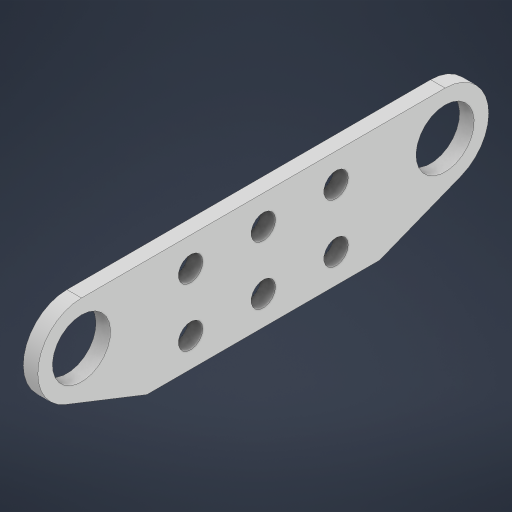
# Autodesk Inventor part: ElevatorCarriageBearingGusset
Saved by Autodesk Inventor 2023 (Build 270158000, 158)
## iProperties
Created: 2023-01-08
Part Number: ElevatorCarriageBearingGusset
Material: Generic
Document SubType Name: Modeling
Designer: Terrence
Density: 1 g/cm^3
Appearance: Default
Author: Terrence
Autodesk Inventor part; units mm, degrees
ref_plane "YZ Plane" through (0, 0, 0) normal (1, 0, 0) x (0, 1, 0)
ref_plane "XZ Plane" through (0, 0, 0) normal (0, 1, 0) x (-1, 0, 0)
ref_plane "XY Plane" through (0, 0, 0) normal (0, 0, 1) x (1, 0, 0)
sketch "Sketch1" plane through (0, 0, 0) normal (1, 0, 0) x (0, 1, 0)
  line L0 (0, 0) -> (25.4, 0)
  line L1 (25.4, 0) -> (25.4, -50.8)
  line L2 (25.4, -50.8) -> (0, -50.8)
  line L3 (0, -50.8) -> (0, 0)
  arc A0 (25.4, 14.2875) -> (7.0144, 17.7826) centre (15.875, 14.2875) ccw
  line L4 (25.4, 0) -> (25.4, 14.2875)
  line L5 (7.0144, 17.7826) -> (0, 0)
  line L6 (15.875, 14.2875) -> (15.875, 0) construction
  circle A1 centre (15.875, 14.2875) radius 14.2875 construction
  line L7 (25.4, -25.4) -> (0, -25.4) construction
  arc A2 (7.0144, -68.5826) -> (25.4, -65.0875) centre (15.875, -65.0875) ccw
  line L8 (25.4, -50.8) -> (25.4, -65.0875)
  line L9 (7.0144, -68.5826) -> (0, -50.8)
  circle A3 centre (15.875, 14.2875) radius 6.35
  circle A4 centre (15.875, -65.0875) radius 6.35
  dimension "d0" = 25.4
  dimension "d1" = 50.8
  dimension "d3" = 19.05
  dimension "d7" = 28.575
  dimension "d8" = 14.2875
  dimension "d11" = 12.7
  constraints: 20 end point, 5 centre point, 4 point on circle, 4 symmetric about line, 2 coincident, 2 midpoint, 2 parallel, 2 perpendicular, 2 tangent, 1 horizontal, 1 point on line, 1 vertical, 2 other
  measures "d0" distance of L1.end L2.end
  measures "d1" distance of L0.end L1.end
  measures "d3" diameter of A0
  measures "d7" diameter of A1
  measures "d8" distance of L6.start L6.end
  measures "d11" diameter of A3
extrude "Extrusion1" add sketch "Sketch1" along normal blind 3.175
sketch "Sketch2" plane through (3.175, 0, 0) normal (1, 0, 0) x (0, 0, -1)
  line L0 (65.0875, 25.4) -> (-14.2875, 25.4) projected
  line L1 (25.4, 25.4) -> (25.4, 0) construction
  line L2 (0, 0) -> (50.8, 0) projected
  line L3 (0, 25.4) -> (50.8, 25.4) construction
  line L4 (50.8, 25.4) -> (50.8, 50.8) construction
  line L5 (50.8, 50.8) -> (0, 50.8) construction
  line L6 (0, 50.8) -> (0, 25.4) construction
  line L7 (3.175, 47.625) -> (47.625, 47.625) construction
  line L8 (47.625, 47.625) -> (47.625, 28.575) construction
  line L9 (47.625, 28.575) -> (3.175, 28.575) construction
  line L10 (3.175, 28.575) -> (3.175, 47.625) construction
  circle A0 centre (9.525, 19.05) radius 2.667
  line L11 (25.4, 12.7) -> (44.9012, 12.7) construction
  circle A1 centre (25.4, 19.05) radius 2.667
  line L12 (9.525, 19.05) -> (32.9122, 19.05) construction
  circle A2 centre (41.275, 19.05) radius 2.667
  circle A3 centre (9.525, 6.35) radius 2.667
  circle A4 centre (25.4, 6.35) radius 2.667
  circle A5 centre (41.275, 6.35) radius 2.667
  dimension "d16" = 50.8
  dimension "d17" = 25.4
  dimension "d18" = 3.175
  dimension "d19" = 5.334
  dimension "d20" = 15.875
  dimension "d21" = 6.35
  dimension "d22" = 5.334
  constraints: 22 end point, 6 centre point, 4 parallel, 4 symmetric about line, 3 horizontal, 3 midpoint, 3 point on line, 2 perpendicular, 7 other
  measures "d16" distance of L4.end L5.end
  measures "d17" distance of L3.end L4.end
  measures "d18" distance between parallel lines of L5 L7
  measures "d19" diameter of A0
  measures "d20" distance from line of L1 L12.start
  measures "d21" distance from line of L0 L12.start
  measures "d22" diameter of A1
extrude "Extrusion2" cut sketch "Sketch2" against normal through all
body "Solid1"
